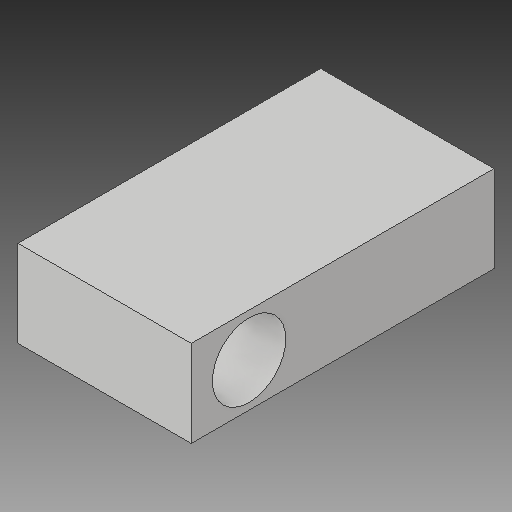
# Autodesk Inventor part: stand2
Saved by Autodesk Inventor 2019 (Build 230136000, 136)
## iProperties
Created: 2019-11-28
Part Number: stand2
Material: Generic
Document SubType Name: Modeling
Designer: felix
Density: 1 g/cm^3
Appearance: Default
Mass: 2472.46 g
Surface Area: 1639.9 cm^2
Volume: 2472.46 cm^3
Author: felix
Autodesk Inventor part; units mm, degrees
ref_plane "YZ Plane" through (0, 0, 0) normal (1, 0, 0) x (0, 1, 0)
ref_plane "XZ Plane" through (0, 0, 0) normal (0, 1, 0) x (-1, 0, 0)
ref_plane "XY Plane" through (0, 0, 0) normal (0, 0, 1) x (1, 0, 0)
sketch "Sketch1" plane through (0, 0, 0) normal (0, 0, 1) x (1, 0, 0)
  line L0 (-150, 75) -> (0, 75)
  line L1 (0, 75) -> (0, 0)
  line L2 (0, 0) -> (-150, 0)
  line L3 (-150, 0) -> (-150, 75)
  dimension "d0" = 150
  dimension "d1" = 75
  constraints: 8 end point, 2 parallel, 1 coincident, 1 horizontal, 1 perpendicular
  measures "d0" distance of L0.start L0.end
  measures "d1" distance of L2.end L0.start
extrude "Extrusion1" add sketch "Sketch1" along normal blind 262
sketch "Sketch2" plane through (0, 0, 0) normal (1, 0, 0) x (0, 0, -1)
  line L0 (-262, 0) -> (-262, 75) projected
  line L1 (0, 75) -> (-262, 75) projected
  point P0 (0, 0)
  point P1 (-212, 37.5)
  dimension "d4" = 50
  dimension "d5" = 37.5
  measures "d4" distance from line of L0 point (-212, 37.5)
  measures "d5" distance from line of L1 point (-212, 37.5)
hole "Hole1" at (0, 37.5, 212) direction (-1, 0, 0) diameter 63.5 end through all
body "Solid1"
